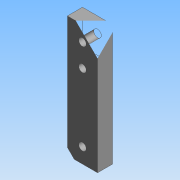
# Autodesk Inventor part: holdersupport
Saved by Autodesk Inventor 2015 (Build 190159000, 159)
## iProperties
Created: 2014-09-02
Part Number: holdersupport
Material: Generic
Document SubType Name: Modeling
Designer: shohei
Density: 1 g/cm^3
Appearance: Default
Author: shohei
Autodesk Inventor part; units mm, degrees
ref_plane "YZ Plane" through (0, 0, 0) normal (1, 0, 0) x (0, 1, 0)
ref_plane "XZ Plane" through (0, 0, 0) normal (0, 1, 0) x (-1, 0, 0)
ref_plane "XY Plane" through (0, 0, 0) normal (0, 0, 1) x (1, 0, 0)
sketch "Sketch4" plane through (0, 0, 0) normal (0, 1, 0) x (-1, 0, 0)
  line L0 (0, 0) -> (20, 0)
  line L1 (20, 0) -> (20, 80)
  line L2 (20, 80) -> (0, 80)
  line L3 (0, 80) -> (0, 0)
  circle A0 centre (-8.1929, 3.0927) radius 2.5
  dimension "d0" = 80
  dimension "d3" = 20
  constraints: 8 end point, 2 parallel, 1 centre point, 1 horizontal, 1 perpendicular
  measures "d0" distance of L0.end L1.end
  measures "d3" distance of L1.end L2.end
extrude "Extrusion1" add sketch "Sketch4" along normal blind 10 contours L3 L2 L1 L0
sketch "Sketch5" plane through (0, 0, 0) normal (0, -1, 0) x (1, 0, 0)
  line L0 (0, 0) -> (-20, 0) projected
  line L1 (0, 80) -> (0, 0) projected
  line L2 (-20, 80) -> (0, 80) projected
  line L3 (-20, 0) -> (-20, 80) projected
  circle A0 centre (-10, 10) radius 2.5
  circle A1 centre (-10, 70) radius 2.5
  circle A2 centre (-10, 55) radius 2.5
  dimension "d5" = 5
  dimension "d6" = 5
  dimension "d7" = 10
  dimension "d8" = 10
  dimension "d9" = 10
  dimension "d10" = 10
  dimension "d13" = 5
  dimension "d17" = 15
  constraints: 3 centre point
  measures "d5" diameter of A0
  measures "d6" diameter of A1
  measures "d7" distance from line of L1 A1.centre
  measures "d8" distance from line of L2 A1.centre
  measures "d9" distance from line of L0 A0.centre
  measures "d10" distance from line of L3 A0.centre
  measures "d13" diameter of A2
  measures "d17" distance of A1.centre A2.centre
extrude "Extrusion3" cut sketch "Sketch5" against normal through all contours A0 | A1 | A2
body "Solid1"
